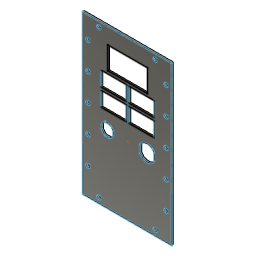
Power Panel v16 (Autodesk Fusion 360 design; units mm, degrees)
Autodesk Fusion 360 part; units mm, degrees
sketch "ControlPanel" plane through (0, 0, 0) normal (0, 1, 0) x (-1, 0, 0)
  line L0 (0, 0) -> (73, 0)
  line L1 (73, 0) -> (73, 41)
  line L2 (73, 41) -> (0, 41)
  line L3 (0, 41) -> (0, 0)
  line L4 (-11.9813, -5) -> (34.0187, -5)
  line L5 (34.0187, -5) -> (34.0187, -32)
  line L6 (34.0187, -32) -> (-11.9813, -32)
  line L7 (-11.9813, -32) -> (-11.9813, -5)
  line L8 (77.6844, -83.0568) -> (77.6844, -82.5327)
  line L9 (-12.1589, -88.0054) -> (-12.1589, -100.8506)
  line L10 (13.8411, -100.8506) -> (13.8411, -88.0054)
  arc A0 (-12.1589, -100.8506) -> (13.8411, -100.8506) centre (0.8411, -94.428) ccw
  arc A1 (13.8411, -88.0054) -> (-12.1589, -88.0054) centre (0.8411, -94.428) ccw
  line L11 (76.8382, -83.928) -> (70.2808, -83.928)
  line L12 (63.0595, -91.1493) -> (63.0595, -97.7068)
  line L13 (70.2808, -104.928) -> (76.8382, -104.928)
  line L14 (84.0595, -97.7068) -> (84.0595, -91.1493)
  arc A2 (70.2808, -83.928) -> (63.0595, -91.1493) centre (73.5595, -94.428) ccw
  arc A3 (84.0595, -91.1493) -> (76.8382, -83.928) centre (73.5595, -94.428) ccw
  arc A4 (63.0595, -97.7068) -> (70.2808, -104.928) centre (73.5595, -94.428) ccw
  arc A5 (76.8382, -104.928) -> (84.0595, -97.7068) centre (73.5595, -94.428) ccw
  line L15 (39.0187, -5) -> (85.0187, -5)
  line L16 (85.0187, -5) -> (85.0187, -32)
  line L17 (85.0187, -32) -> (39.0187, -32)
  line L18 (39.0187, -32) -> (39.0187, -5)
  line L19 (-11.9813, -37) -> (34.0187, -37)
  line L20 (34.0187, -37) -> (34.0187, -64)
  line L21 (34.0187, -64) -> (-11.9813, -64)
  line L22 (-11.9813, -64) -> (-11.9813, -37)
  line L23 (39.0187, -37) -> (85.0187, -37)
  line L24 (85.0187, -37) -> (85.0187, -64)
  line L25 (85.0187, -64) -> (39.0187, -64)
  line L26 (39.0187, -64) -> (39.0187, -37)
  line L27 (34.0187, -5) -> (39.0187, -5) construction
  circle A6 centre (36.5, -94.428) radius 0.6723 construction
  line L28 (119.0595, -139.428) -> (119.0595, 71) construction
  line L29 (119.0595, 71) -> (-44.1589, 71) construction
  line L30 (-44.1589, 71) -> (-44.1589, -139.428) construction
  line L31 (-44.1589, 71) -> (119.0595, 71)
  line L32 (119.0595, 71) -> (119.0595, -219)
  line L33 (119.0595, -219) -> (-44.1589, -219)
  line L34 (-44.1589, -219) -> (-44.1589, 71)
  circle A7 centre (-14.1589, 61) radius 3
  circle A8 centre (89.0595, 61) radius 3
  circle A9 centre (-34.1589, 31) radius 3
  circle A10 centre (109.0551, 31) radius 3
  circle A11 centre (-34.1589, -19) radius 3
  circle A12 centre (109.0551, -19) radius 3
  circle A13 centre (-34.1589, -69) radius 3
  circle A14 centre (109.0551, -69) radius 3
  circle A15 centre (-34.1589, -119) radius 3
  circle A16 centre (109.0551, -119) radius 3
  circle A17 centre (-34.1589, -169) radius 3
  circle A18 centre (109.0551, -169) radius 3
  circle A19 centre (-14.1589, -209) radius 3
  circle A20 centre (89.0595, -209) radius 3
  point P0 (73.5595, -94.428)
  point P1 (0.8411, -94.428)
  point P2 (73.5595, -94.428)
  point P3 (0.8411, -94.428)
  point P4 (73.5595, -94.428)
  point P5 (-14.1589, -209)
  point P6 (89.0595, -209)
  dimension "d12" = 73
  dimension "d13" = 41
  dimension "d15" = 46
  dimension "d16" = 27
  dimension "d17" = 5
  dimension "d33" = 29
  dimension "d36" = 22
  dimension "d88" = 46
  dimension "d89" = 27
  dimension "d90" = 5
  dimension "d91" = 46
  dimension "d92" = 27
  dimension "d93" = 5
  dimension "d94" = 46
  dimension "d95" = 27
  dimension "d96" = 5
  dimension "d110" = 210.428
  dimension "d111" = 290
  dimension "d113" = 6
  dimension "d114" = 30
  dimension "d115" = 6
  dimension "d116" = 30
  dimension "d123" = 6
  dimension "d124" = 40
  dimension "d127" = 143.214
  dimension "d128" = -200
  constraint horizontal L0
  constraint vertical L1
  constraint horizontal L2
  constraint vertical L3
  constraint coincident L0.start L3.end
  constraint horizontal L4
  constraint vertical L5
  constraint horizontal L6
  constraint vertical L7
  constraint coincident P3 P1
  constraint parallel L9 L10
  constraint concentric A0 A1
  constraint horizontal L11
  constraint perpendicular L11 L12
  constraint parallel L11 L13
  constraint parallel L12 L14
  constraint concentric A2 A4
  constraint coincident L14.end A4
  constraint concentric A3 A4
  constraint coincident L13.end A4
  constraint concentric A4 A5
  constraint horizontal L15
  constraint vertical L16
  constraint horizontal L17
  constraint vertical L18
  constraint horizontal L19
  constraint vertical L20
  constraint horizontal L21
  constraint vertical L22
  constraint collinear L7 L22
  constraint horizontal L23
  constraint vertical L24
  constraint horizontal L25
  constraint vertical L26
  constraint collinear L18 L26
  constraint collinear L19 L23
  constraint horizontal L31
  constraint vertical L32
  constraint horizontal L33
  constraint vertical L34
  measures "d12" distance of L0.start L0.end
  measures "d13" distance of L0.start L2.end
  measures "d15" distance of L4.start L4.end
  measures "d16" distance of L4.start L6.end L0.start
  measures "d17" distance of L0 L4
  measures "d33" diameter of A0
  measures "d36" diameter of A2
  measures "d88" distance of L15.start L15.end
  measures "d89" distance of L15.start L17.end
  measures "d90" distance of L0 L15
  measures "d91" distance of L19.start L19.end
  measures "d92" distance of L19.start L21.end
  measures "d93" distance of L6 L19
  measures "d94" distance of L23.start L23.end
  measures "d95" distance of L23.start L25.end
  measures "d96" distance of L5 L18
  measures "d110" distance of L28.start L28.end
  measures "d111" distance of L29.end L33.end
  measures "d113" diameter of A7
  measures "d114" distance of L34 A7.centre
  measures "d115" diameter of A8
  measures "d116" distance of L28 A8.centre
  measures "d123" diameter of A9
  measures "d124" distance of L31 A9.centre
extrude "Extrude3" add sketch "ControlPanel" along normal blind 3 contours L31 L32 L33 L34 | A19 | A20
extrude "Extrude5" cut sketch "ControlPanel" along normal mid plane 12 contours A19
extrude "Extrude6" cut sketch "ControlPanel" along normal mid plane 12 contours A20
extrude "Extrude1" [suppressed]
equation "m2_w = 73 mm"
equation "m2_h = 41 mm"
equation "m1_w = 46 mm"
equation "m1_h = 27 mm"
equation "mpwr_dia = 12.2 mm"
equation "mpwr_key = 1 mm"
equation "reset_dia = 12.5 mm"
equation "apwr_dia = 29 mm"
equation "apwr_key = 26 mm"
equation "estop_dia = 22 mm"
equation "estop_key = 21 mm"
equation "d12 = m2_w"
equation "d13 = m2_h"
equation "meter_v = 5 mm"
equation "d15 = m1_w"
equation "d16 = m1_h"
equation "d17 = meter_v"
equation "apwr_shell = 37 mm"
equation "botrow_offset = 35 mm"
equation "d33 = apwr_dia"
equation "d36 = estop_dia"
equation "sw_dist = 100 mm"
equation "sw_offs = 25 mm"
equation "text_top_offs = 5 mm"
equation "d88 = m1_w"
equation "d89 = m1_h"
equation "d90 = meter_v"
equation "d91 = m1_w"
equation "d92 = m1_h"
equation "d93 = meter_v"
equation "d94 = m1_w"
equation "d95 = m1_h"
